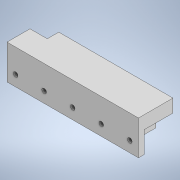
# Autodesk Inventor part: side_bumper
Saved by Autodesk Inventor 2020 (Build 240168000, 168)
## iProperties
Created: 2022-07-15
Part Number: side_bumper
Material: 일반
Document SubType Name: Modeling
Designer: SeungJin
Density: 1 g/cm^3
Appearance: 기본값
Author: SeungJin
Autodesk Inventor part; units mm, degrees
ref_plane "YZ Plane" through (0, 0, 0) normal (1, 0, 0) x (0, 1, 0)
ref_plane "XZ Plane" through (0, 0, 0) normal (0, 1, 0) x (-1, 0, 0)
ref_plane "XY Plane" through (0, 0, 0) normal (0, 0, 1) x (1, 0, 0)
sketch "스케치1" plane through (0, 0, 0) normal (0, 0, 1) x (1, 0, 0)
  line L0 (6, 0) -> (18, 0) projected
  line L1 (6, 0) -> (6, -540) projected
  line L2 (18, -540) -> (6, -540) projected
  line L3 (18, 0) -> (18, -540) projected
  line L4 (-12, 0) -> (0, 0) projected
  line L5 (-12, 0) -> (-12, -540) projected
  line L6 (0, -540) -> (-12, -540) projected
  line L7 (0, 0) -> (0, -540) projected
  line L8 (18, 22.5444) -> (18, 12.5098) projected
  line L9 (18, 12.5098) -> (18, -220) projected
  line L10 (-192.5399, 0) -> (-180.5399, 0) projected
  line L11 (-192.5399, 0) -> (-192.5399, -540) projected
  line L12 (-180.5399, -540) -> (-192.5399, -540) projected
  line L13 (-180.5399, 0) -> (-180.5399, -540) projected
  line L14 (-210.5399, 0) -> (-198.5399, 0) projected
  line L15 (-210.5399, 0) -> (-210.5399, -540) projected
  line L16 (-198.5399, -540) -> (-210.5399, -540) projected
  line L17 (-198.5399, 0) -> (-198.5399, -540) projected
  line L18 (18, 22.5444) -> (-210.5399, 22.5444)
  line L19 (-210.5399, 22.5444) -> (-210.5399, -37.4556)
  line L20 (-210.5399, -37.4556) -> (18, -37.4556)
  line L21 (18, -37.4556) -> (18, 22.5444)
  line L22 (18, 12.5444) -> (-210.5399, 12.5444)
  dimension "d0" = 60
  dimension "d1" = 10
  constraints: 10 end point, 3 point on line, 2 parallel, 2 perpendicular, 1 horizontal
  measures "d0" distance of L19.end L18.end
  measures "d1" distance between parallel lines of L22 L18
extrude "돌출1" add sketch "스케치1" along normal blind 10 and the other way blind 50 contours L22 L19 L18 L8
sketch "스케치2" plane through (-210.5399, 22.5444, 10) normal (0, 1, 0) x (1, 0, 0)
  line L0 (0, 60) -> (0, 0) projected
  line L1 (228.5399, 0) -> (0, 0) projected
  line L2 (228.5399, 60) -> (228.5399, 0) projected
  line L3 (0, 60) -> (228.5399, 60) projected
  circle A0 centre (-63.5, 111.3) radius 75.8469 projected
  line L4 (-155.5399, 160) -> (-155.5399, 55) projected
  line L5 (-139.3469, 111.3) -> (-155.5399, 111.3)
  line L6 (0, 0) -> (228.5399, 0) projected
  line L7 (30, 0) -> (30, 60)
  line L8 (0, 60) -> (0, 0) projected
  line L9 (30, 0) -> (0, 0)
  line L10 (0, 0) -> (0, 40)
  line L11 (0, 40) -> (30, 40)
  line L12 (30, 40) -> (30, 0)
  point P0 (210.5399, 10)
  point P1 (30, 40)
  dimension "d7" = 16.193
  dimension "d8" = 40
  dimension "d44" = 30
  constraints: 12 end point, 4 point on line, 3 perpendicular, 2 parallel, 1 horizontal, 1 horizontal alignment, 1 other
  measures "d7" distance of L5.start L5.end
  measures "d8" distance of L9.end L10.end
  measures "d44" distance between parallel lines of L7 L0
extrude "돌출2" cut sketch "스케치2" against normal through all contours L3 L7 L11 L0
ref_plane "작업 평면1" through (-180.5399, 0, 0) normal (0, 0, 1) x (1, 0, 0)
sketch "스케치3" plane through (-180.5399, 0, 0) normal (0, 0, 1) x (1, 0, 0)
  line L0 (-30, 22.5444) -> (-30, 12.5444) projected
  line L1 (-30, 12.5444) -> (198.5399, 12.5444) projected
  line L2 (198.5399, 12.5444) -> (198.5399, 22.5444) projected
  line L3 (198.5399, 22.5444) -> (-30, 22.5444) projected
  line L4 (-30, 12.5444) -> (198.5399, 12.5444) projected
  line L5 (-30, 0) -> (-18, 0) projected
  line L6 (-30, 0) -> (-30, -540) projected
  line L7 (-18, -540) -> (-30, -540) projected
  line L8 (-18, 0) -> (-18, -540) projected
  line L9 (-12, 0) -> (0, 0) projected
  line L10 (-12, 0) -> (-12, -540) projected
  line L11 (0, -540) -> (-12, -540) projected
  line L12 (0, 0) -> (0, -540) projected
  line L13 (168.5399, 0) -> (180.5399, 0) projected
  line L14 (168.5399, 0) -> (168.5399, -540) projected
  line L15 (180.5399, -540) -> (168.5399, -540) projected
  line L16 (180.5399, 0) -> (180.5399, -540) projected
  line L17 (186.5399, 0) -> (198.5399, 0) projected
  line L18 (186.5399, 0) -> (186.5399, -540) projected
  line L19 (198.5399, -540) -> (186.5399, -540) projected
  line L20 (198.5399, 0) -> (198.5399, -540) projected
  line L21 (198.5399, 12.5444) -> (-30, 12.5444)
  line L22 (-30, 12.5444) -> (-30, -37.4556)
  line L23 (-30, -37.4556) -> (198.5399, -37.4556)
  line L24 (198.5399, -37.4556) -> (198.5399, 12.5444)
  dimension "d11" = 50
  constraints: 8 end point, 2 parallel, 1 horizontal, 1 perpendicular, 1 point on line
  measures "d11" distance of L22.end L21.end
extrude "돌출3" add sketch "스케치3" along normal blind 10 contours L1 L24 L17 L18 L23 L16 L13 L14 L12 L9 L10 L8 L5 L22 | L5 L8 L23 L6 | L20 L23 L18 L17 | L10 L9 L12 L23 | L23 L14 L13 L16
ref_plane "작업 평면2" through (-12, -260, -30) normal (0, 0, -1) x (0, 1, 0)
sketch "스케치4" plane through (-180.5399, 0, 0) normal (0, 0, -1) x (-1, 0, 0)
  line L0 (-180.5399, -260) -> (-168.5399, -260)
  line L1 (-168.5399, 0) -> (-168.5399, -260)
  line L2 (-180.5399, 0) -> (-168.5399, 0)
  line L3 (-180.5399, 0) -> (-180.5399, -260)
  line L4 (-198.5399, -260) -> (-186.5399, -260)
  line L5 (-186.5399, 0) -> (-186.5399, -260)
  line L6 (-198.5399, 0) -> (-186.5399, 0)
  line L7 (-198.5399, 0) -> (-198.5399, -260)
  line L8 (0, 12.5444) -> (0, 22.5444)
  line L9 (0, 22.5444) -> (-198.5399, 22.5444)
  line L10 (-198.5399, 22.5444) -> (-198.5399, 12.5444)
  line L11 (-198.5399, 12.5444) -> (0, 12.5444)
  line L12 (30, 12.5444) -> (0, 12.5444)
  line L13 (30, 22.5444) -> (30, 12.5444)
  line L14 (0, 22.5444) -> (30, 22.5444)
  line L15 (0, 22.5444) -> (0, 12.5444)
  line L16 (18, -260) -> (30, -260)
  line L17 (30, 0) -> (30, -260)
  line L18 (18, 0) -> (30, 0)
  line L19 (18, 0) -> (18, -260)
  line L20 (0, -260) -> (12, -260)
  line L21 (12, 0) -> (12, -260)
  line L22 (0, 0) -> (12, 0)
  line L23 (0, 0) -> (0, -260)
  line L24 (-198.5399, 0) -> (30, 0)
  line L25 (30, 0) -> (30, 12.5444)
  line L26 (30, 12.5444) -> (-198.5399, 12.5444)
  line L27 (-198.5399, 12.5444) -> (-198.5399, 0)
  line L28 (30, 12.5444) -> (30, -37.4556)
  line L29 (-198.5399, 12.5444) -> (30, 12.5444)
  line L30 (-198.5399, -37.4556) -> (-198.5399, 12.5444)
  line L31 (30, -37.4556) -> (-198.5399, -37.4556)
  line L32 (-198.5399, 0) -> (30, 0)
  line L33 (30, 0) -> (30, -37.4556)
  line L34 (30, -37.4556) -> (-198.5399, -37.4556)
  line L35 (-198.5399, -37.4556) -> (-198.5399, 0)
  line L36 (30, -37.4556) -> (-198.5399, -37.4556)
  line L37 (-99.27, 0) -> (-69.27, 0)
  line L38 (-69.27, 0) -> (-69.27, -37.4556)
  line L39 (-69.27, -37.4556) -> (-99.27, -37.4556)
  line L40 (-99.27, -37.4556) -> (-99.27, 0)
  line L41 (-99.27, 0) -> (-69.27, -37.4556) construction
  line L42 (-69.27, 0) -> (-99.27, -37.4556) construction
  line L43 (0, 0) -> (0, 12.5444)
  point P0 (0, 12.5444)
  point P1 (-84.27, -18.7278)
  point P2 (0, -37.4556)
  point P3 (-168.5399, -37.4556)
extrude "돌출4" add sketch "스케치4" along normal blind 50 contours L1 L24 L40 L31 | L24 L6 L27 L11 L43 L2 | L38 L24 L23 L31
ref_plane "작업 평면3" through (-210.5399, 20.5444, 10) normal (0, 1, 0) x (1, 0, 0)
sketch "스케치7" plane through (-180.5399, 0, 0) normal (0, 0, -1) x (-1, 0, 0)
  line L0 (0, -260) -> (12, -260) projected
  line L1 (12, 0) -> (12, -260) projected
  line L2 (0, 0) -> (12, 0) projected
  line L3 (0, 0) -> (0, -260) projected
  line L4 (18, -260) -> (30, -260) projected
  line L5 (30, 0) -> (30, -260) projected
  line L6 (18, 0) -> (30, 0) projected
  line L7 (18, 0) -> (18, -260) projected
  line L8 (30, 12.5444) -> (0, 12.5444) projected
  line L9 (30, 22.5444) -> (30, 12.5444) projected
  line L10 (0, 22.5444) -> (30, 22.5444) projected
  line L11 (0, 22.5444) -> (0, 12.5444) projected
  line L12 (-198.5399, 12.5444) -> (0, 12.5444) projected
  line L13 (0, 12.5444) -> (30, 12.5444)
  line L14 (30, 12.5444) -> (30, 0)
  line L15 (30, 0) -> (0, 0)
  line L16 (0, 0) -> (0, 12.5444)
  point P0 (-180.5399, 0)
  constraints: 8 end point, 2 parallel, 1 horizontal, 1 perpendicular
extrude "돌출7" add sketch "스케치7" along normal blind 30 contours L16 L8 L14 L6 L15 L2
sketch "스케치12" plane through (0, 0, 10) normal (0, 0, 1) x (1, 0, 0)
  line L0 (-180.5399, -37.4556) -> (-180.5399, 22.5444) projected
  line L1 (-180.5399, 22.5444) -> (18, 22.5444) projected
  line L2 (18, 22.5444) -> (18, 0) projected
  line L3 (18, 0) -> (-12, 0) projected
  line L4 (-12, 0) -> (-12, -37.4556) projected
  line L5 (-12, -37.4556) -> (-81.27, -37.4556) projected
  line L6 (-81.27, -37.4556) -> (-81.27, 0) projected
  line L7 (-81.27, 0) -> (-111.27, 0) projected
  line L8 (-111.27, 0) -> (-111.27, -37.4556) projected
  line L9 (-111.27, -37.4556) -> (-180.5399, -37.4556) projected
  line L10 (-180.5399, 0) -> (-12, 0)
  point P0 (0, 0)
  point P1 (-145.9049, -18.7278)
  point P2 (-46.635, -18.7278)
  constraints: 2 end point, 1 horizontal, 1 point on line
hole "구멍1" at (-145.9049, -18.7278, 10) at (-46.635, -18.7278, 10) direction (0, 0, -1) diameter 4.5 end through all counterbore diameter 8 counterbore depth 40 clearance for "Hex Head Cap Screw ISO 24017" size "M4" standard "ISO"
sketch "스케치13" plane through (0, 0, 10) normal (0, 0, 1) x (1, 0, 0)
  line L0 (-81.27, 0) -> (-81.27, -37.4556) projected
  line L1 (-111.27, -37.4556) -> (-111.27, 0) projected
  line L2 (-180.5399, 0) -> (-180.5399, -37.4556) projected
  line L3 (-12, -37.4556) -> (-12, 0) projected
  line L4 (-111.27, 0) -> (-81.27, 0) projected
  line L5 (-12, 0) -> (18, 0) projected
  line L6 (-210.5399, 0) -> (-180.5399, 0) projected
  point P0 (0, 0)
  point P1 (-195.5399, -18.7278)
  point P2 (-96.27, -18.7278)
  point P3 (3, -18.7278)
hole "구멍2" at (-195.5399, -18.7278, 10) at (-96.27, -18.7278, 10) at (3, -18.7278, 10) direction (0, 0, -1) diameter 4.5 end through all counterbore diameter 8 counterbore depth 5 clearance for "Hex Head Cap Screw ISO 24017" size "M4" standard "ISO"
